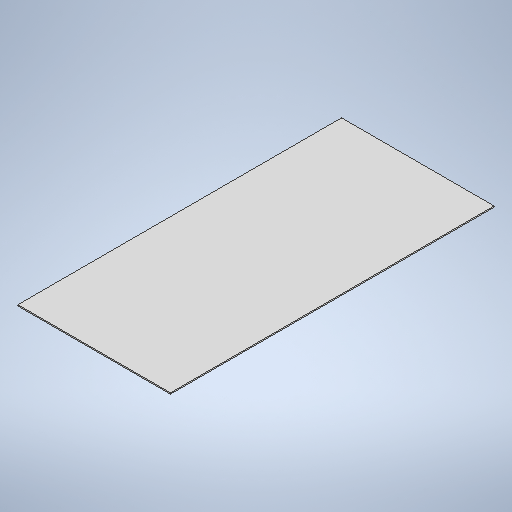
# Autodesk Inventor part: final
Saved by Autodesk Inventor 2025.2 (Build 292293000, 293)
## iProperties
Created: 2025-05-26
Part Number: final
Material: Generic
Document SubType Name: Sheet Metal
Designer: abdal
Density: 1 g/cm^3
Sheet Metal Rule: Default_mm
Appearance: Default
Author: abdal
Autodesk Inventor part; units mm, degrees
ref_plane "YZ Plane" through (0, 0, 0) normal (1, 0, 0) x (0, 1, 0)
ref_plane "XZ Plane" through (0, 0, 0) normal (0, 1, 0) x (-1, 0, 0)
ref_plane "XY Plane" through (0, 0, 0) normal (0, 0, 1) x (1, 0, 0)
sketch "Sketch1" plane through (0, 0, 0) normal (0, 1, 0) x (-1, 0, 0)
  line L0 (130, 275.75) -> (-130, 275.75)
  line L1 (-130, 275.75) -> (-130, -275.75)
  line L2 (-130, -275.75) -> (130, -275.75)
  line L3 (130, -275.75) -> (130, 275.75)
  line L4 (130, 275.75) -> (-130, -275.75) construction
  line L5 (-130, 275.75) -> (130, -275.75) construction
  point P0 (0, 0)
  dimension "d0" = 551.5
  dimension "d1" = 260
  measures "d0" distance of L2.end L0.start
  measures "d1" distance of L1.end L2.end
extrude "Plate1" add sketch "Sketch1" along normal blind 2
equation "\"d2\" = Thickness"
equation "\"BendRadius\" = Thickness"
equation "\"BendReliefWidth\" = Thickness"
equation "\"BendReliefDepth\" = 0.5 * Thickness"
equation "\"CornerReliefSize\" = 4 * Thickness"
equation "\"MinimumRemnant\" = 2 * Thickness"
equation "\"TransitionRadius\" = BendRadius"
equation "\"JacobiRadiusSize\" = BendRadius"
equation "\"GapSize\" = Thickness"
equation "\"Thickness\" = 2"
body "Solid1"
